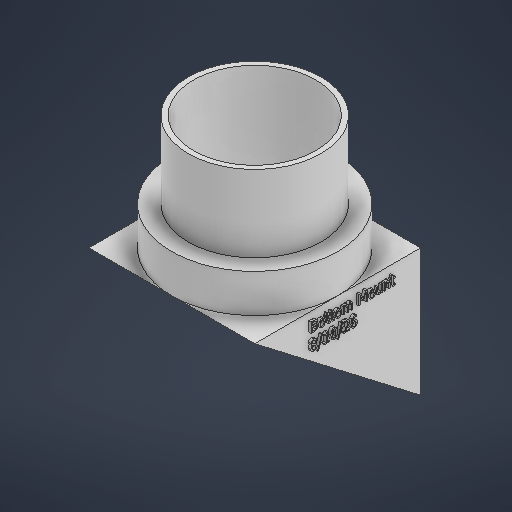
# Autodesk Inventor part: cam_bottom_mount
Saved by Autodesk Inventor 2027 (Build 310192060, 192F)
## iProperties
Created: 2026-07-30
Part Number: cam_bottom_mount
Material: Generic
Document SubType Name: Modeling
Designer: farde
Density: 1 g/cm^3
Appearance: Default
Author: farde
Autodesk Inventor part; units mm, degrees
ref_plane "YZ Plane" through (0, 0, 0) normal (1, 0, 0) x (0, 1, 0)
ref_plane "XZ Plane" through (0, 0, 0) normal (0, 1, 0) x (-1, 0, 0)
ref_plane "XY Plane" through (0, 0, 0) normal (0, 0, 1) x (1, 0, 0)
sketch "Sketch1" plane through (0, 0, 0) normal (0, 1, 0) x (-1, 0, 0)
  circle A0 centre (0, 0) radius 26
  dimension "d0" = 52
  constraints: 1 centre point, 1 coincident
  measures "d0" diameter of A0
extrude "Extrusion1" add sketch "Sketch1" along normal blind 30
sketch "Sketch2" plane through (0, 0, 0) normal (0, -1, 0) x (1, 0, 0)
  circle A0 centre (0, 0) radius 32.5
  dimension "d3" = 65
  constraints: 1 centre point, 1 coincident
  measures "d3" diameter of A0
extrude "Extrusion2" add sketch "Sketch2" along normal blind 15
sketch "Sketch3" plane through (0, 30, 0) normal (0, 1, 0) x (1, 0, 0)
  circle A0 centre (0, 0) radius 24
  dimension "d6" = 48
  constraints: 1 centre point, 1 coincident
  measures "d6" diameter of A0
extrude "Extrusion3" cut sketch "Sketch3" against normal blind 214.475
sketch "Sketch4" plane through (0, -15, 0) normal (0, -1, 0) x (1, 0, 0)
  point P0 (0, 0)
sketch "Sketch7" plane through (0, -15, 0) normal (0, -1, 0) x (1, 0, 0)
  line L0 (32.5, -32.5) -> (-32.5, -32.5)
  line L1 (-32.5, -32.5) -> (-32.5, 32.5)
  line L2 (-32.5, 32.5) -> (32.5, 32.5)
  line L3 (32.5, 32.5) -> (32.5, -32.5)
  line L4 (32.5, -32.5) -> (-32.5, 32.5) construction
  line L5 (-32.5, -32.5) -> (32.5, 32.5) construction
  point P0 (0, 0)
  dimension "d14" = 65
  dimension "d15" = 65
  constraints: 12 end point, 2 midpoint, 2 parallel, 1 horizontal, 1 perpendicular
  measures "d14" distance of L0.end L1.end
  measures "d15" distance of L1.end L2.end
extrude "Extrusion6" add sketch "Sketch7" along normal blind 50
sketch "Sketch8" plane through (0, -65, 0) normal (0, -1, 0) x (1, 0, 0)
  line L0 (-28.5, 28.5) -> (28.5, 28.5)
  line L1 (28.5, 28.5) -> (28.5, -28.5)
  line L2 (28.5, -28.5) -> (-28.5, -28.5)
  line L3 (-28.5, -28.5) -> (-28.5, 28.5)
  line L4 (-28.5, 28.5) -> (28.5, -28.5) construction
  line L5 (28.5, 28.5) -> (-28.5, -28.5) construction
  point P0 (0, 0)
  dimension "d18" = 57
  dimension "d19" = 57
  constraints: 12 end point, 2 midpoint, 2 parallel, 1 horizontal, 1 perpendicular
  measures "d18" distance of L1.end L2.end
  measures "d19" distance of L0.end L1.end
extrude "Extrusion7" cut sketch "Sketch8" against normal blind 47.5
sketch "Sketch9" plane through (32.5, -15, -12.5) normal (1, 0, 0) x (0, 0, -1)
  line L0 (20, -50) -> (-45, -50) projected
  line L1 (-45, 0) -> (-45, -50) projected
  line L2 (20, -50) -> (-45, 0)
  line L3 (-45, 0) -> (-45, -50)
  line L4 (-41, -50) -> (-41, -2.5) projected
  line L5 (-45, -50) -> (20, -50)
  point P0 (-12.5, 15)
  constraints: 6 end point, 1 parallel, 1 perpendicular
extrude "Extrusion8" cut sketch "Sketch9" against normal blind 89.6875
sketch "Sketch10" plane through (0, -17.5, 0) normal (0, -1, 0) x (1, 0, 0)
  circle A0 centre (0, 0) radius 5
  dimension "d24" = 10
  constraints: 1 centre point, 1 coincident
  measures "d24" diameter of A0
extrude "Extrusion9" cut sketch "Sketch10" against normal blind 12.9125
sketch "Sketch11" plane through (-12.5, -15, -32.5) normal (0, 0, -1) x (-1, 0, 0)
  circle A0 centre (-12.5, -24.4758) radius 5
  point P0 (-12.5, 15)
  dimension "d27" = 10
  constraints: 1 centre point
  measures "d27" diameter of A0
extrude "Extrusion10" cut sketch "Sketch11" against normal blind 74.7375
sketch "Sketch12" plane through (-28.5, -17.5, -28.5) normal (0, 0, 1) x (1, 0, 0)
  circle A0 centre (28.5, -21.9741) radius 9.5
  point P0 (28.5, 17.5)
  dimension "d31" = 19
  constraints: 1 centre point
  measures "d31" diameter of A0
extrude "Extrusion11" cut sketch "Sketch12" against normal blind 1
sketch "Sketch13" plane through (32.5, -15, 0) normal (1, 0, 0) x (0, 0, -1)
  line L0 (-11.7103, -2.766) -> (44.5294, -2.766) construction
  line L1 (44.5294, -2.766) -> (44.5294, -13.0987) construction
  line L2 (44.5294, -13.0987) -> (-11.7103, -13.0987) construction
  line L3 (-11.7103, -13.0987) -> (-11.7103, -2.766) construction
  spline S0 degree 2 poles (-8.6878, -5.4522) (-8.6878, -5.7413) (-8.9078, -6.1843) (-9.09, -6.3288) knots 0 0 0 1 2 2 2
  spline S1 degree 2 poles (-9.09, -6.3288) (-9.3099, -6.4985) (-9.8095, -6.643) (-10.2054, -6.643) knots 0 0 0 1 2 2 2
  line L4 (-10.2054, -6.643) -> (-11.3176, -6.643)
  line L5 (-11.3176, -6.643) -> (-11.3176, -2.766)
  line L6 (-11.3176, -2.766) -> (-10.2902, -2.766)
  spline S2 degree 2 poles (-10.2902, -2.766) (-9.8755, -2.766) (-9.4607, -2.8194) (-9.2722, -2.923) knots 0 0 0 1 2 2 2
  spline S3 degree 2 poles (-9.2722, -2.923) (-9.0617, -3.033) (-8.8701, -3.3943) (-8.8701, -3.6394) knots 0 0 0 1 2 2 2
  spline S4 degree 2 poles (-8.8701, -3.6394) (-8.8701, -3.9127) (-9.1591, -4.3463) (-9.4136, -4.4688) knots 0 0 0 1 2 2 2
  line L7 (-9.4136, -4.4688) -> (-9.4136, -4.4877)
  spline S5 degree 2 poles (-9.4136, -4.4877) (-9.068, -4.5819) (-8.6878, -5.0815) (-8.6878, -5.4522) knots 0 0 0 1 2 2 2
  spline S6 degree 2 poles (-9.2251, -5.4742) (-9.2251, -5.2543) (-9.3508, -4.9715) (-9.5393, -4.871) knots 0 0 0 1 2 2 2
  spline S7 degree 2 poles (-9.5393, -4.871) (-9.6618, -4.8082) (-9.9509, -4.7705) (-10.2179, -4.7705) knots 0 0 0 1 2 2 2
  line L8 (-10.2179, -4.7705) -> (-10.8023, -4.7705)
  line L9 (-10.8023, -4.7705) -> (-10.8023, -6.2031)
  line L10 (-10.8023, -6.2031) -> (-10.3844, -6.2031)
  spline S8 degree 2 poles (-10.3844, -6.2031) (-10.0451, -6.2031) (-9.6555, -6.1403) (-9.5047, -6.0398) knots 0 0 0 1 2 2 2
  spline S9 degree 2 poles (-9.5047, -6.0398) (-9.3602, -5.9361) (-9.2251, -5.6785) (-9.2251, -5.4742) knots 0 0 0 1 2 2 2
  spline S10 degree 2 poles (-9.4073, -3.7117) (-9.4073, -3.5734) (-9.5016, -3.366) (-9.6053, -3.3064) knots 0 0 0 1 2 2 2
  spline S11 degree 2 poles (-9.6053, -3.3064) (-9.7309, -3.2372) (-10.0357, -3.2058) (-10.309, -3.2058) knots 0 0 0 1 2 2 2
  line L11 (-10.309, -3.2058) -> (-10.8023, -3.2058)
  line L12 (-10.8023, -3.2058) -> (-10.8023, -4.34)
  line L13 (-10.8023, -4.34) -> (-10.2179, -4.34)
  spline S12 degree 2 poles (-10.2179, -4.34) (-9.976, -4.34) (-9.7467, -4.2898) (-9.6241, -4.2112) knots 0 0 0 1 2 2 2
  spline S13 degree 2 poles (-9.6241, -4.2112) (-9.5047, -4.1358) (-9.4073, -3.8939) (-9.4073, -3.7117) knots 0 0 0 1 2 2 2
  spline S14 degree 2 poles (-5.8225, -5.1883) (-5.8225, -5.9235) (-6.5294, -6.7247) (-7.1201, -6.7247) knots 0 0 0 1 2 2 2
  spline S15 degree 2 poles (-7.1201, -6.7247) (-7.7264, -6.7247) (-8.4208, -5.8984) (-8.4208, -5.1883) knots 0 0 0 1 2 2 2
  spline S16 degree 2 poles (-8.4208, -5.1883) (-8.4208, -4.4594) (-7.7044, -3.652) (-7.1201, -3.652) knots 0 0 0 1 2 2 2
  spline S17 degree 2 poles (-7.1201, -3.652) (-6.5294, -3.652) (-5.8225, -4.4563) (-5.8225, -5.1883) knots 0 0 0 1 2 2 2
  spline S18 degree 2 poles (-6.3283, -5.1883) (-6.3283, -4.6228) (-6.7399, -4.073) (-7.1201, -4.073) knots 0 0 0 1 2 2 2
  spline S19 degree 2 poles (-7.1201, -4.073) (-7.5002, -4.073) (-7.9149, -4.6228) (-7.9149, -5.1883) knots 0 0 0 1 2 2 2
  spline S20 degree 2 poles (-7.9149, -5.1883) (-7.9149, -5.7382) (-7.5002, -6.3037) (-7.1201, -6.3037) knots 0 0 0 1 2 2 2
  spline S21 degree 2 poles (-7.1201, -6.3037) (-6.743, -6.3037) (-6.3283, -5.7476) (-6.3283, -5.1883) knots 0 0 0 1 2 2 2
  spline S22 degree 2 poles (-4.44, -6.6996) (-4.8391, -6.6996) (-5.2884, -6.244) (-5.2884, -5.7507) knots 0 0 0 1 2 2 2
  line L14 (-5.2884, -5.7507) -> (-5.2884, -4.1389)
  line L15 (-5.2884, -4.1389) -> (-5.6182, -4.1389)
  line L16 (-5.6182, -4.1389) -> (-5.6182, -3.7336)
  line L17 (-5.6182, -3.7336) -> (-5.2884, -3.7336)
  line L18 (-5.2884, -3.7336) -> (-5.2884, -2.8979)
  line L19 (-5.2884, -2.8979) -> (-4.7982, -2.8979)
  line L20 (-4.7982, -2.8979) -> (-4.7982, -3.7336)
  line L21 (-4.7982, -3.7336) -> (-3.8965, -3.7336)
  line L22 (-3.8965, -3.7336) -> (-3.8965, -4.1389)
  line L23 (-3.8965, -4.1389) -> (-4.7982, -4.1389)
  line L24 (-4.7982, -4.1389) -> (-4.7982, -5.5245)
  spline S23 degree 2 poles (-4.7982, -5.5245) (-4.7982, -5.7444) (-4.7825, -5.9864) (-4.7291, -6.09) knots 0 0 0 1 2 2 2
  spline S24 degree 2 poles (-4.7291, -6.09) (-4.6851, -6.1812) (-4.4872, -6.2723) (-4.3175, -6.2723) knots 0 0 0 1 2 2 2
  spline S25 degree 2 poles (-4.3175, -6.2723) (-4.1981, -6.2723) (-3.9751, -6.2) (-3.9248, -6.178) knots 0 0 0 1 2 2 2
  line L25 (-3.9248, -6.178) -> (-3.8965, -6.178)
  line L26 (-3.8965, -6.178) -> (-3.8965, -6.6179)
  spline S26 degree 2 poles (-3.8965, -6.6179) (-4.0347, -6.6556) (-4.3175, -6.6996) (-4.44, -6.6996) knots 0 0 0 1 2 2 2
  spline S27 degree 2 poles (-2.6555, -6.6996) (-3.0545, -6.6996) (-3.5038, -6.244) (-3.5038, -5.7507) knots 0 0 0 1 2 2 2
  line L27 (-3.5038, -5.7507) -> (-3.5038, -4.1389)
  line L28 (-3.5038, -4.1389) -> (-3.8337, -4.1389)
  line L29 (-3.8337, -4.1389) -> (-3.8337, -3.7336)
  line L30 (-3.8337, -3.7336) -> (-3.5038, -3.7336)
  line L31 (-3.5038, -3.7336) -> (-3.5038, -2.8979)
  line L32 (-3.5038, -2.8979) -> (-3.0136, -2.8979)
  line L33 (-3.0136, -2.8979) -> (-3.0136, -3.7336)
  line L34 (-3.0136, -3.7336) -> (-2.1119, -3.7336)
  line L35 (-2.1119, -3.7336) -> (-2.1119, -4.1389)
  line L36 (-2.1119, -4.1389) -> (-3.0136, -4.1389)
  line L37 (-3.0136, -4.1389) -> (-3.0136, -5.5245)
  spline S28 degree 2 poles (-3.0136, -5.5245) (-3.0136, -5.7444) (-2.9979, -5.9864) (-2.9445, -6.09) knots 0 0 0 1 2 2 2
  spline S29 degree 2 poles (-2.9445, -6.09) (-2.9005, -6.1812) (-2.7026, -6.2723) (-2.5329, -6.2723) knots 0 0 0 1 2 2 2
  spline S30 degree 2 poles (-2.5329, -6.2723) (-2.4135, -6.2723) (-2.1905, -6.2) (-2.1402, -6.178) knots 0 0 0 1 2 2 2
  line L38 (-2.1402, -6.178) -> (-2.1119, -6.178)
  line L39 (-2.1119, -6.178) -> (-2.1119, -6.6179)
  spline S31 degree 2 poles (-2.1119, -6.6179) (-2.2502, -6.6556) (-2.5329, -6.6996) (-2.6555, -6.6996) knots 0 0 0 1 2 2 2
  spline S32 degree 2 poles (0.6403, -5.1883) (0.6403, -5.9235) (-0.0666, -6.7247) (-0.6572, -6.7247) knots 0 0 0 1 2 2 2
  spline S33 degree 2 poles (-0.6572, -6.7247) (-1.2636, -6.7247) (-1.958, -5.8984) (-1.958, -5.1883) knots 0 0 0 1 2 2 2
  spline S34 degree 2 poles (-1.958, -5.1883) (-1.958, -4.4594) (-1.2416, -3.652) (-0.6572, -3.652) knots 0 0 0 1 2 2 2
  spline S35 degree 2 poles (-0.6572, -3.652) (-0.0666, -3.652) (0.6403, -4.4563) (0.6403, -5.1883) knots 0 0 0 1 2 2 2
  spline S36 degree 2 poles (0.1345, -5.1883) (0.1345, -4.6228) (-0.2771, -4.073) (-0.6572, -4.073) knots 0 0 0 1 2 2 2
  spline S37 degree 2 poles (-0.6572, -4.073) (-1.0374, -4.073) (-1.4521, -4.6228) (-1.4521, -5.1883) knots 0 0 0 1 2 2 2
  spline S38 degree 2 poles (-1.4521, -5.1883) (-1.4521, -5.7382) (-1.0374, -6.3037) (-0.6572, -6.3037) knots 0 0 0 1 2 2 2
  spline S39 degree 2 poles (-0.6572, -6.3037) (-0.2802, -6.3037) (0.1345, -5.7476) (0.1345, -5.1883) knots 0 0 0 1 2 2 2
  line L40 (4.442, -6.643) -> (4.442, -4.959)
  spline S40 degree 2 poles (4.442, -4.959) (4.442, -4.7579) (4.4106, -4.4154) (4.3603, -4.3212) knots 0 0 0 1 2 2 2
  spline S41 degree 2 poles (4.3603, -4.3212) (4.31, -4.2175) (4.1184, -4.117) (3.9519, -4.117) knots 0 0 0 1 2 2 2
  spline S42 degree 2 poles (3.9519, -4.117) (3.8011, -4.117) (3.4554, -4.3023) (3.2732, -4.4783) knots 0 0 0 1 2 2 2
  spline S43 degree 2 poles (3.2732, -4.4783) (3.2764, -4.5223) (3.2826, -4.6448) (3.2826, -4.7265) knots 0 0 0 1 2 2 2
  line L41 (3.2826, -4.7265) -> (3.2826, -6.643)
  line L42 (3.2826, -6.643) -> (2.7925, -6.643)
  line L43 (2.7925, -6.643) -> (2.7925, -4.959)
  spline S44 degree 2 poles (2.7925, -4.959) (2.7925, -4.7579) (2.7611, -4.4154) (2.7108, -4.3212) knots 0 0 0 1 2 2 2
  spline S45 degree 2 poles (2.7108, -4.3212) (2.6606, -4.2175) (2.4689, -4.117) (2.3024, -4.117) knots 0 0 0 1 2 2 2
  spline S46 degree 2 poles (2.3024, -4.117) (2.1453, -4.117) (1.7965, -4.3149) (1.6332, -4.4688) knots 0 0 0 1 2 2 2
  line L44 (1.6332, -4.4688) -> (1.6332, -6.643)
  line L45 (1.6332, -6.643) -> (1.143, -6.643)
  line L46 (1.143, -6.643) -> (1.143, -3.7336)
  line L47 (1.143, -3.7336) -> (1.6332, -3.7336)
  line L48 (1.6332, -3.7336) -> (1.6332, -4.0541)
  spline S47 degree 2 poles (1.6332, -4.0541) (1.8248, -3.8625) (2.2018, -3.652) (2.4281, -3.652) knots 0 0 0 1 2 2 2
  spline S48 degree 2 poles (2.4281, -3.652) (2.6857, -3.652) (3.0847, -3.8876) (3.1884, -4.1547) knots 0 0 0 1 2 2 2
  spline S49 degree 2 poles (3.1884, -4.1547) (3.4115, -3.9064) (3.8325, -3.652) (4.0775, -3.652) knots 0 0 0 1 2 2 2
  spline S50 degree 2 poles (4.0775, -3.652) (4.266, -3.652) (4.5739, -3.7682) (4.6871, -3.9002) knots 0 0 0 1 2 2 2
  spline S51 degree 2 poles (4.6871, -3.9002) (4.8033, -4.0321) (4.9321, -4.428) (4.9321, -4.7265) knots 0 0 0 1 2 2 2
  line L49 (4.9321, -4.7265) -> (4.9321, -6.643)
  line L50 (4.9321, -6.643) -> (4.442, -6.643)
  line L51 (10.6472, -6.643) -> (10.1319, -6.643)
  line L52 (10.1319, -6.643) -> (10.1319, -3.3032)
  line L53 (10.1319, -3.3032) -> (9.1202, -5.5748)
  line L54 (9.1202, -5.5748) -> (8.806, -5.5748)
  line L55 (8.806, -5.5748) -> (7.8038, -3.3032)
  line L56 (7.8038, -3.3032) -> (7.8038, -6.643)
  line L57 (7.8038, -6.643) -> (7.3231, -6.643)
  line L58 (7.3231, -6.643) -> (7.3231, -2.766)
  line L59 (7.3231, -2.766) -> (8.0269, -2.766)
  line L60 (8.0269, -2.766) -> (8.9945, -4.9244)
  line L61 (8.9945, -4.9244) -> (9.9308, -2.766)
  line L62 (9.9308, -2.766) -> (10.6472, -2.766)
  line L63 (10.6472, -2.766) -> (10.6472, -6.643)
  spline S52 degree 2 poles (13.7859, -5.1883) (13.7859, -5.9235) (13.079, -6.7247) (12.4883, -6.7247) knots 0 0 0 1 2 2 2
  spline S53 degree 2 poles (12.4883, -6.7247) (11.8819, -6.7247) (11.1876, -5.8984) (11.1876, -5.1883) knots 0 0 0 1 2 2 2
  spline S54 degree 2 poles (11.1876, -5.1883) (11.1876, -4.4594) (11.9039, -3.652) (12.4883, -3.652) knots 0 0 0 1 2 2 2
  spline S55 degree 2 poles (12.4883, -3.652) (13.079, -3.652) (13.7859, -4.4563) (13.7859, -5.1883) knots 0 0 0 1 2 2 2
  spline S56 degree 2 poles (13.28, -5.1883) (13.28, -4.6228) (12.8685, -4.073) (12.4883, -4.073) knots 0 0 0 1 2 2 2
  spline S57 degree 2 poles (12.4883, -4.073) (12.1081, -4.073) (11.6934, -4.6228) (11.6934, -5.1883) knots 0 0 0 1 2 2 2
  spline S58 degree 2 poles (11.6934, -5.1883) (11.6934, -5.7382) (12.1081, -6.3037) (12.4883, -6.3037) knots 0 0 0 1 2 2 2
  spline S59 degree 2 poles (12.4883, -6.3037) (12.8653, -6.3037) (13.28, -5.7476) (13.28, -5.1883) knots 0 0 0 1 2 2 2
  line L64 (16.5507, -6.643) -> (16.0606, -6.643)
  line L65 (16.0606, -6.643) -> (16.0606, -6.3225)
  spline S60 degree 2 poles (16.0606, -6.3225) (15.8344, -6.5205) (15.4291, -6.7247) (15.1777, -6.7247) knots 0 0 0 1 2 2 2
  spline S61 degree 2 poles (15.1777, -6.7247) (14.9892, -6.7247) (14.653, -6.599) (14.5305, -6.4639) knots 0 0 0 1 2 2 2
  spline S62 degree 2 poles (14.5305, -6.4639) (14.4048, -6.3288) (14.2666, -5.9172) (14.2666, -5.6219) knots 0 0 0 1 2 2 2
  line L66 (14.2666, -5.6219) -> (14.2666, -3.7336)
  line L67 (14.2666, -3.7336) -> (14.7567, -3.7336)
  line L68 (14.7567, -3.7336) -> (14.7567, -5.3925)
  spline S63 degree 2 poles (14.7567, -5.3925) (14.7567, -5.625) (14.7913, -5.9298) (14.851, -6.0429) knots 0 0 0 1 2 2 2
  spline S64 degree 2 poles (14.851, -6.0429) (14.9107, -6.156) (15.1149, -6.2597) (15.3065, -6.2597) knots 0 0 0 1 2 2 2
  spline S65 degree 2 poles (15.3065, -6.2597) (15.4856, -6.2597) (15.8909, -6.0555) (16.0606, -5.9078) knots 0 0 0 1 2 2 2
  line L69 (16.0606, -5.9078) -> (16.0606, -3.7336)
  line L70 (16.0606, -3.7336) -> (16.5507, -3.7336)
  line L71 (16.5507, -3.7336) -> (16.5507, -6.643)
  line L72 (19.5449, -6.643) -> (19.0548, -6.643)
  line L73 (19.0548, -6.643) -> (19.0548, -4.9841)
  spline S66 degree 2 poles (19.0548, -4.9841) (19.0548, -4.783) (19.0171, -4.4374) (18.9605, -4.3337) knots 0 0 0 1 2 2 2
  spline S67 degree 2 poles (18.9605, -4.3337) (18.9008, -4.2238) (18.6872, -4.117) (18.505, -4.117) knots 0 0 0 1 2 2 2
  spline S68 degree 2 poles (18.505, -4.117) (18.3227, -4.117) (17.9363, -4.3117) (17.7509, -4.4688) knots 0 0 0 1 2 2 2
  line L74 (17.7509, -4.4688) -> (17.7509, -6.643)
  line L75 (17.7509, -6.643) -> (17.2608, -6.643)
  line L76 (17.2608, -6.643) -> (17.2608, -3.7336)
  line L77 (17.2608, -3.7336) -> (17.7509, -3.7336)
  line L78 (17.7509, -3.7336) -> (17.7509, -4.0573)
  spline S69 degree 2 poles (17.7509, -4.0573) (17.9708, -3.8593) (18.395, -3.652) (18.6338, -3.652) knots 0 0 0 1 2 2 2
  spline S70 degree 2 poles (18.6338, -3.652) (19.0611, -3.652) (19.5449, -4.2175) (19.5449, -4.7548) knots 0 0 0 1 2 2 2
  line L79 (19.5449, -4.7548) -> (19.5449, -6.643)
  spline S71 degree 2 poles (21.1127, -6.6996) (20.7137, -6.6996) (20.2644, -6.244) (20.2644, -5.7507) knots 0 0 0 1 2 2 2
  line L80 (20.2644, -5.7507) -> (20.2644, -4.1389)
  line L81 (20.2644, -4.1389) -> (19.9345, -4.1389)
  line L82 (19.9345, -4.1389) -> (19.9345, -3.7336)
  line L83 (19.9345, -3.7336) -> (20.2644, -3.7336)
  line L84 (20.2644, -3.7336) -> (20.2644, -2.8979)
  line L85 (20.2644, -2.8979) -> (20.7545, -2.8979)
  line L86 (20.7545, -2.8979) -> (20.7545, -3.7336)
  line L87 (20.7545, -3.7336) -> (21.6562, -3.7336)
  line L88 (21.6562, -3.7336) -> (21.6562, -4.1389)
  line L89 (21.6562, -4.1389) -> (20.7545, -4.1389)
  line L90 (20.7545, -4.1389) -> (20.7545, -5.5245)
  spline S72 degree 2 poles (20.7545, -5.5245) (20.7545, -5.7444) (20.7702, -5.9864) (20.8237, -6.09) knots 0 0 0 1 2 2 2
  spline S73 degree 2 poles (20.8237, -6.09) (20.8676, -6.1812) (21.0656, -6.2723) (21.2352, -6.2723) knots 0 0 0 1 2 2 2
  spline S74 degree 2 poles (21.2352, -6.2723) (21.3546, -6.2723) (21.5777, -6.2) (21.628, -6.178) knots 0 0 0 1 2 2 2
  line L91 (21.628, -6.178) -> (21.6562, -6.178)
  line L92 (21.6562, -6.178) -> (21.6562, -6.6179)
  spline S75 degree 2 poles (21.6562, -6.6179) (21.518, -6.6556) (21.2352, -6.6996) (21.1127, -6.6996) knots 0 0 0 1 2 2 2
  spline S76 degree 2 poles (-10.2556, -13.1145) (-10.5447, -13.1145) (-11.0191, -12.9416) (-11.1856, -12.7814) knots 0 0 0 1 2 2 2
  spline S77 degree 2 poles (-11.1856, -12.7814) (-11.349, -12.6243) (-11.5187, -12.197) (-11.5187, -11.9551) knots 0 0 0 1 2 2 2
  spline S78 degree 2 poles (-11.5187, -11.9551) (-11.5187, -11.6409) (-11.1825, -11.1131) (-10.862, -10.956) knots 0 0 0 1 2 2 2
  line L93 (-10.862, -10.956) -> (-10.862, -10.9403)
  spline S79 degree 2 poles (-10.862, -10.9403) (-11.1479, -10.7738) (-11.4244, -10.3779) (-11.4244, -10.0826) knots 0 0 0 1 2 2 2
  spline S80 degree 2 poles (-11.4244, -10.0826) (-11.4244, -9.6458) (-10.7646, -9.0615) (-10.2556, -9.0615) knots 0 0 0 1 2 2 2
  spline S81 degree 2 poles (-10.2556, -9.0615) (-9.7278, -9.0615) (-9.09, -9.6144) (-9.09, -10.048) knots 0 0 0 1 2 2 2
  spline S82 degree 2 poles (-9.09, -10.048) (-9.09, -10.3088) (-9.3948, -10.8178) (-9.6807, -10.9623) knots 0 0 0 1 2 2 2
  line L94 (-9.6807, -10.9623) -> (-9.6807, -10.978)
  spline S83 degree 2 poles (-9.6807, -10.978) (-9.3414, -11.1351) (-8.9926, -11.5875) (-8.9926, -11.9457) knots 0 0 0 1 2 2 2
  spline S84 degree 2 poles (-8.9926, -11.9457) (-8.9926, -12.4421) (-9.7152, -13.1145) (-10.2556, -13.1145) knots 0 0 0 1 2 2 2
  spline S85 degree 2 poles (-9.5267, -11.9959) (-9.5267, -11.7572) (-9.7152, -11.4744) (-9.9823, -11.3299) knots 0 0 0 1 2 2 2
  spline S86 degree 2 poles (-9.9823, -11.3299) (-10.0703, -11.2796) (-10.3656, -11.1634) (-10.551, -11.088) knots 0 0 0 1 2 2 2
  spline S87 degree 2 poles (-10.551, -11.088) (-10.7646, -11.2293) (-10.994, -11.6503) (-10.994, -11.9174) knots 0 0 0 1 2 2 2
  spline S88 degree 2 poles (-10.994, -11.9174) (-10.994, -12.2693) (-10.5698, -12.728) (-10.2493, -12.728) knots 0 0 0 1 2 2 2
  spline S89 degree 2 poles (-10.2493, -12.728) (-9.9226, -12.728) (-9.5267, -12.3353) (-9.5267, -11.9959) knots 0 0 0 1 2 2 2
  spline S90 degree 2 poles (-9.599, -10.0543) (-9.599, -9.7935) (-9.9477, -9.4448) (-10.2588, -9.4448) knots 0 0 0 1 2 2 2
  spline S91 degree 2 poles (-10.2588, -9.4448) (-10.5415, -9.4448) (-10.9029, -9.7558) (-10.9029, -10.0229) knots 0 0 0 1 2 2 2
  spline S92 degree 2 poles (-10.9029, -10.0229) (-10.9029, -10.2145) (-10.7175, -10.4816) (-10.5321, -10.5884) knots 0 0 0 1 2 2 2
  spline S93 degree 2 poles (-10.5321, -10.5884) (-10.4536, -10.6324) (-10.1205, -10.7863) (-9.9854, -10.8303) knots 0 0 0 1 2 2 2
  spline S94 degree 2 poles (-9.9854, -10.8303) (-9.7592, -10.6575) (-9.599, -10.2899) (-9.599, -10.0543) knots 0 0 0 1 2 2 2
  line L95 (-6.9064, -8.9766) -> (-8.4239, -13.8685)
  line L96 (-8.4239, -13.8685) -> (-8.8638, -13.8685)
  line L97 (-8.8638, -13.8685) -> (-7.3526, -8.9766)
  line L98 (-7.3526, -8.9766) -> (-6.9064, -8.9766)
  line L99 (-4.283, -13.0265) -> (-6.1744, -13.0265)
  line L100 (-6.1744, -13.0265) -> (-6.1744, -12.6306)
  line L101 (-6.1744, -12.6306) -> (-5.4706, -12.6306)
  line L102 (-5.4706, -12.6306) -> (-5.4706, -10.0323)
  line L103 (-5.4706, -10.0323) -> (-6.1744, -10.0323)
  line L104 (-6.1744, -10.0323) -> (-6.1744, -9.6773)
  spline S95 degree 2 poles (-6.1744, -9.6773) (-5.7753, -9.6773) (-5.3983, -9.451) (-5.3732, -9.1369) knots 0 0 0 1 2 2 2
  line L105 (-5.3732, -9.1369) -> (-4.971, -9.1369)
  line L106 (-4.971, -9.1369) -> (-4.971, -12.6306)
  line L107 (-4.971, -12.6306) -> (-4.283, -12.6306)
  line L108 (-4.283, -12.6306) -> (-4.283, -13.0265)
  spline S96 degree 2 poles (-1.1568, -11.088) (-1.1568, -12.131) (-1.7632, -13.1082) (-2.3947, -13.1082) knots 0 0 0 1 2 2 2
  spline S97 degree 2 poles (-2.3947, -13.1082) (-3.0356, -13.1082) (-3.6357, -12.1122) (-3.6357, -11.0911) knots 0 0 0 1 2 2 2
  spline S98 degree 2 poles (-3.6357, -11.0911) (-3.6357, -10.0417) (-3.0294, -9.0709) (-2.3947, -9.0709) knots 0 0 0 1 2 2 2
  spline S99 degree 2 poles (-2.3947, -9.0709) (-1.7569, -9.0709) (-1.1568, -10.0763) (-1.1568, -11.088) knots 0 0 0 1 2 2 2
  spline S100 degree 2 poles (-1.8229, -12.2693) (-1.7475, -12.0776) (-1.6846, -11.487) (-1.6846, -11.088) knots 0 0 0 1 2 2 2
  spline S101 degree 2 poles (-1.6846, -11.088) (-1.6846, -10.6889) (-1.7475, -10.1014) (-1.826, -9.9035) knots 0 0 0 1 2 2 2
  spline S102 degree 2 poles (-1.826, -9.9035) (-1.9046, -9.7055) (-2.1779, -9.5013) (-2.3947, -9.5013) knots 0 0 0 1 2 2 2
  spline S103 degree 2 poles (-2.3947, -9.5013) (-2.6115, -9.5013) (-2.8911, -9.7055) (-2.9728, -9.9098) knots 0 0 0 1 2 2 2
  spline S104 degree 2 poles (-2.9728, -9.9098) (-3.0513, -10.1077) (-3.1079, -10.7109) (-3.1079, -11.0911) knots 0 0 0 1 2 2 2
  spline S105 degree 2 poles (-3.1079, -11.0911) (-3.1079, -11.4995) (-3.0576, -12.0462) (-2.9759, -12.2599) knots 0 0 0 1 2 2 2
  spline S106 degree 2 poles (-2.9759, -12.2599) (-2.9005, -12.4609) (-2.6209, -12.6777) (-2.3947, -12.6777) knots 0 0 0 1 2 2 2
  spline S107 degree 2 poles (-2.3947, -12.6777) (-2.1811, -12.6777) (-1.9014, -12.4735) (-1.8229, -12.2693) knots 0 0 0 1 2 2 2
  line L109 (0.9514, -8.9766) -> (-0.5661, -13.8685)
  line L110 (-0.5661, -13.8685) -> (-1.006, -13.8685)
  line L111 (-1.006, -13.8685) -> (0.5052, -8.9766)
  line L112 (0.5052, -8.9766) -> (0.9514, -8.9766)
  line L113 (3.7696, -13.0265) -> (1.3787, -13.0265)
  line L114 (1.3787, -13.0265) -> (1.3787, -12.4767)
  spline S108 degree 2 poles (1.3787, -12.4767) (1.6363, -12.2347) (2.095, -11.7854) (2.315, -11.5435) knots 0 0 0 1 2 2 2
  spline S109 degree 2 poles (2.315, -11.5435) (2.758, -11.0565) (3.0816, -10.4721) (3.0816, -10.1611) knots 0 0 0 1 2 2 2
  spline S110 degree 2 poles (3.0816, -10.1611) (3.0816, -9.9977) (2.981, -9.7527) (2.8899, -9.6741) knots 0 0 0 1 2 2 2
  spline S111 degree 2 poles (2.8899, -9.6741) (2.7988, -9.5956) (2.56, -9.517) (2.4155, -9.517) knots 0 0 0 1 2 2 2
  spline S112 degree 2 poles (2.4155, -9.517) (2.2772, -9.517) (1.9945, -9.5861) (1.8657, -9.6396) knots 0 0 0 1 2 2 2
  spline S113 degree 2 poles (1.8657, -9.6396) (1.7557, -9.6835) (1.5515, -9.8092) (1.4886, -9.8532) knots 0 0 0 1 2 2 2
  line L115 (1.4886, -9.8532) -> (1.4604, -9.8532)
  line L116 (1.4604, -9.8532) -> (1.4604, -9.3002)
  spline S114 degree 2 poles (1.4604, -9.3002) (1.6206, -9.2217) (2.1956, -9.0677) (2.4532, -9.0677) knots 0 0 0 1 2 2 2
  spline S115 degree 2 poles (2.4532, -9.0677) (2.9967, -9.0677) (3.6094, -9.6427) (3.6094, -10.1328) knots 0 0 0 1 2 2 2
  spline S116 degree 2 poles (3.6094, -10.1328) (3.6094, -10.3622) (3.5026, -10.7455) (3.4083, -10.9089) knots 0 0 0 1 2 2 2
  spline S117 degree 2 poles (3.4083, -10.9089) (3.3141, -11.0785) (3.0407, -11.4116) (2.8899, -11.5718) knots 0 0 0 1 2 2 2
  spline S118 degree 2 poles (2.8899, -11.5718) (2.6448, -11.8389) (2.0448, -12.4107) (1.8657, -12.5772) knots 0 0 0 1 2 2 2
  line L117 (1.8657, -12.5772) -> (3.7696, -12.5772)
  line L118 (3.7696, -12.5772) -> (3.7696, -13.0265)
  spline S119 degree 2 poles (6.7387, -11.7697) (6.7387, -12.0682) (6.5408, -12.5741) (6.3742, -12.7437) knots 0 0 0 1 2 2 2
  spline S120 degree 2 poles (6.3742, -12.7437) (6.2014, -12.9228) (5.7679, -13.1082) (5.5071, -13.1082) knots 0 0 0 1 2 2 2
  spline S121 degree 2 poles (5.5071, -13.1082) (5.2463, -13.1082) (4.8159, -12.9322) (4.6525, -12.7563) knots 0 0 0 1 2 2 2
  spline S122 degree 2 poles (4.6525, -12.7563) (4.4514, -12.5458) (4.2252, -11.8389) (4.2252, -11.3236) knots 0 0 0 1 2 2 2
  spline S123 degree 2 poles (4.2252, -11.3236) (4.2252, -10.8178) (4.4326, -10.004) (4.6494, -9.7024) knots 0 0 0 1 2 2 2
  spline S124 degree 2 poles (4.6494, -9.7024) (4.8599, -9.4071) (5.5259, -9.0772) (5.9627, -9.0772) knots 0 0 0 1 2 2 2
  spline S125 degree 2 poles (5.9627, -9.0772) (6.0915, -9.0772) (6.3177, -9.1023) (6.4025, -9.1306) knots 0 0 0 1 2 2 2
  line L119 (6.4025, -9.1306) -> (6.4025, -9.6301)
  line L120 (6.4025, -9.6301) -> (6.3805, -9.6301)
  spline S126 degree 2 poles (6.3805, -9.6301) (6.3083, -9.5924) (6.0443, -9.5264) (5.8935, -9.5264) knots 0 0 0 1 2 2 2
  spline S127 degree 2 poles (5.8935, -9.5264) (5.4097, -9.5264) (4.8159, -10.18) (4.7593, -10.8209) knots 0 0 0 1 2 2 2
  spline S128 degree 2 poles (4.7593, -10.8209) (4.9447, -10.6921) (5.3343, -10.5507) (5.5668, -10.5507) knots 0 0 0 1 2 2 2
  spline S129 degree 2 poles (5.5668, -10.5507) (5.793, -10.5507) (6.1323, -10.6418) (6.3177, -10.78) knots 0 0 0 1 2 2 2
  spline S130 degree 2 poles (6.3177, -10.78) (6.5313, -10.9403) (6.7387, -11.4367) (6.7387, -11.7697) knots 0 0 0 1 2 2 2
  spline S131 degree 2 poles (6.2109, -11.7917) (6.2109, -11.5529) (6.0852, -11.2293) (5.9469, -11.1162) knots 0 0 0 1 2 2 2
  spline S132 degree 2 poles (5.9469, -11.1162) (5.8433, -11.0345) (5.5856, -10.9811) (5.4505, -10.9811) knots 0 0 0 1 2 2 2
  spline S133 degree 2 poles (5.4505, -10.9811) (5.2683, -10.9811) (4.9258, -11.0911) (4.7593, -11.1948) knots 0 0 0 1 2 2 2
  spline S134 degree 2 poles (4.7593, -11.1948) (4.7562, -11.2513) (4.7499, -11.3582) (4.7499, -11.4398) knots 0 0 0 1 2 2 2
  spline S135 degree 2 poles (4.7499, -11.4398) (4.7499, -11.842) (4.907, -12.3353) (5.0264, -12.4641) knots 0 0 0 1 2 2 2
  spline S136 degree 2 poles (5.0264, -12.4641) (5.1363, -12.5866) (5.3751, -12.684) (5.5102, -12.684) knots 0 0 0 1 2 2 2
  spline S137 degree 2 poles (5.5102, -12.684) (5.8244, -12.684) (6.2109, -12.2379) (6.2109, -11.7917) knots 0 0 0 1 2 2 2
  point P0 (0, 15)
  constraints: 2 other
emboss "Emboss1" sketch "Sketch13" operation add depth 1 direction (-1, 0, 0)
body "Solid1"
